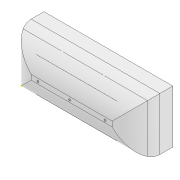
# Autodesk Inventor part: DeckelKoch
Saved by Autodesk Inventor 2020 (Build 240168000, 168)
## iProperties
Created: 2022-01-25
Part Number: DeckelKoch
Material: Polyaryletherketon-Kunststoff
Document SubType Name: Modeling
Designer: Julian Uhl
Density: 1.32 g/cm^3
Appearance: Glatt - Weiß
Author: Julian Uhl
Autodesk Inventor part; units mm, degrees
ref_plane "YZ Plane" through (0, 0, 0) normal (1, 0, 0) x (0, 1, 0)
ref_plane "XZ Plane" through (0, 0, 0) normal (0, 1, 0) x (-1, 0, 0)
ref_plane "XY Plane" through (0, 0, 0) normal (0, 0, 1) x (1, 0, 0)
sketch "Skizze1" plane through (0, 0, 0) normal (0, 0, 1) x (1, 0, 0)
  line L0 (-56, 0) -> (336, 0) projected
  line L1 (0, -23) -> (0, 138) projected
  line L2 (0, 0) -> (280, 0)
  line L3 (280, 0) -> (280, 115)
  line L4 (280, 115) -> (0, 115)
  line L5 (0, 115) -> (0, 0)
  line L6 (5, 110) -> (275, 110)
  line L7 (275, 110) -> (275, 5)
  line L8 (275, 5) -> (5, 5)
  line L9 (5, 5) -> (5, 110)
  point P0 (0, 115)
  dimension "d0" = 280
  dimension "d1" = 115
  dimension "d2" = 5
  dimension "d3" = 5
  dimension "d4" = 5
  dimension "d5" = 5
  constraints: 16 end point, 4 parallel, 2 horizontal, 2 perpendicular
  measures "d0" distance between parallel lines of L3 L1
  measures "d1" distance between parallel lines of L0 L4
  measures "d2" distance between parallel lines of L4 L6
  measures "d3" distance between parallel lines of L3 L7
  measures "d4" distance between parallel lines of L2 L8
  measures "d5" distance between parallel lines of L5 L9
extrude "Extrusion1" add sketch "Skizze1" along normal blind 50
sketch "Skizze2" plane through (0, 0, 50) normal (0, 0, 1) x (1, 0, 0)
  point P0 (0, 0)
sketch "Skizze3" plane through (0, 0, 50) normal (0, 0, 1) x (1, 0, 0)
  line L0 (0, 115) -> (0, 0) projected
  line L1 (0, 0) -> (280, 0) projected
  line L2 (0, 115) -> (280, 115)
  line L3 (280, 115) -> (280, 0)
  line L4 (280, 0) -> (0, 0)
  line L5 (0, 0) -> (0, 115)
  line L6 (280, 115) -> (0, 115) projected
  line L7 (280, 0) -> (0, 0)
  line L8 (0, 0) -> (0, 115)
  line L9 (0, 115) -> (280, 115)
  line L10 (280, 115) -> (280, 0)
  constraints: 16 end point, 4 parallel, 2 horizontal, 2 perpendicular
extrude "Extrusion2" add sketch "Skizze3" along normal blind 30
fillet "Rundung1" radius 52 4 edges at (140, 115, 80) (140, 0, 80) (0, 57.5, 80) (280, 57.5, 80)
sketch "Skizze5" plane through (0, 0, 0) normal (0, 0, -1) x (-1, 0, 0)
  line L0 (-5, 110) -> (-275, 110) projected
  line L1 (-182.5, 110) -> (-182.5, 5)
  line L2 (-275, 5) -> (-5, 5) projected
  line L3 (-92.5, 110) -> (-92.5, 5)
  line L4 (-275, 110) -> (-275, 5) projected
  line L5 (-177.5, 110) -> (-177.5, 5)
  line L6 (-87.5, 110) -> (-87.5, 5)
  point P0 (0, 0)
  dimension "d11" = 92.5
  dimension "d12" = 182.5
  dimension "d13" = 5
  dimension "d14" = 5
  constraints: 8 end point, 8 point on line, 2 perpendicular, 1 parallel, 1 vertical
  measures "d11" distance between parallel lines of L1 L4
  measures "d12" distance between parallel lines of L3 L4
  measures "d13" distance between parallel lines of L5 L1
  measures "d14" distance between parallel lines of L6 L3
extrude "Extrusion3" add sketch "Skizze5" against normal blind 50 contours L6 L2 L3 L0 | L5 L2 L1 L0
sketch "Skizze6" plane through (0, 0, 80) normal (0, 0, 1) x (1, 0, 0)
  line L0 (52, 52) -> (52, 63) projected
  line L1 (228, 63) -> (228, 52) projected
  line L2 (177.5, 110) -> (177.5, 5) projected
  line L3 (52, 63) -> (228, 63) projected
  point P0 (0, 0)
  point P1 (67, 57)
  point P2 (136, 57)
  point P3 (213, 57)
  dimension "d17" = 15
  dimension "d18" = 15
  dimension "d19" = 41.5
  dimension "d20" = 6
  dimension "d21" = 6
  dimension "d22" = 6
  measures "d17" distance from line of point (67, 57) L0
  measures "d18" distance from line of L1 point (213, 57)
  measures "d19" distance from line of L2 point (136, 57)
  measures "d20" distance from line of L3 point (67, 57)
  measures "d21" distance from line of L3 point (136, 57)
  measures "d22" distance from line of L3 point (213, 57)
hole "Bohrung1" at (67, 57, 80) at (136, 57, 80) at (213, 57, 80) direction (0, 0, -1) diameter 4 end through all
sketch "Skizze8" plane through (0, 0, 50) normal (0, 0, -1) x (-1, 0, 0)
  line L0 (-52, 95) -> (-228, 95)
  line L1 (-228, 95) -> (-228, 20)
  line L2 (-228, 20) -> (-52, 20)
  line L3 (-52, 20) -> (-52, 95)
  line L4 (-228, 63) -> (-228, 52) projected
  line L5 (-52, 52) -> (-52, 63) projected
  line L6 (-92.5, 110) -> (-177.5, 110) projected
  line L7 (-177.5, 5) -> (-92.5, 5) projected
  point P0 (0, 0)
  dimension "d30" = 0
  dimension "d31" = 0
  dimension "d32" = 15
  dimension "d33" = 15
  constraints: 8 end point, 2 parallel, 1 horizontal, 1 perpendicular
  measures "d30" distance between parallel lines of L1 L4
  measures "d31" distance between parallel lines of L5 L3
  measures "d32" distance between parallel lines of L6 L0
  measures "d33" distance between parallel lines of L7 L2
extrude "Extrusion4" cut sketch "Skizze8" against normal blind 19
